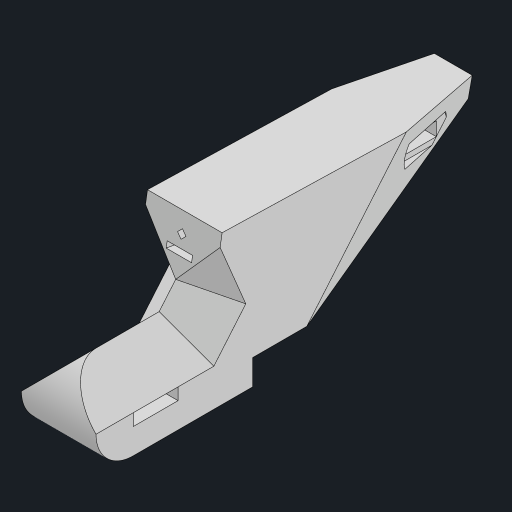
# Autodesk Inventor part: om_Body_2.0
Saved by Autodesk Inventor 2023 (Build 270158000, 158)
## iProperties
Created: 2022-06-16
Part Number: om_Body_2.0
Material: 一般
Document SubType Name: Modeling
Designer: legot
Density: 1 g/cm^3
Appearance: 既定
Mass: 644.355 g
Surface Area: 645.321 cm^2
Volume: 644.355 cm^3
Author: legot
Autodesk Inventor part; units mm, degrees
ref_plane "YZ Plane" through (0, 0, 0) normal (1, 0, 0) x (0, 1, 0)
ref_plane "XZ Plane" through (0, 0, 0) normal (0, 1, 0) x (-1, 0, 0)
ref_plane "XY Plane" through (0, 0, 0) normal (0, 0, 1) x (1, 0, 0)
sketch "スケッチ1" plane through (0, 0, 0) normal (1, 0, 0) x (0, 1, 0)
  line L0 (-36.4926, 6.1068) -> (-49.6929, 17.1832)
  line L1 (-49.6929, 17.1832) -> (-49.6929, 84.5055)
  arc A0 (-74.6929, 84.5055) -> (-99.6929, 59.5055) centre (-74.6929, 59.5055) ccw
  line L2 (-99.6929, 59.5055) -> (-99.6929, -20.4945)
  line L3 (-82.6929, -56.7945) -> (-19.7119, -179.9383)
  line L4 (-19.7119, -179.9383) -> (-4.7119, -179.9383)
  line L5 (-4.7119, -179.9383) -> (0, 0)
  line L6 (0, 0) -> (0, -120.6859) construction
  line L7 (-36.4926, 6.1068) -> (0, 0)
  line L8 (0, 0) -> (23.9477, 0) construction
  line L9 (0.4951, 2.9589) -> (52.2751, -5.7061)
  line L10 (52.2751, -5.7061) -> (51.78, -8.665)
  line L11 (51.78, -8.665) -> (0, 0)
  line L12 (39.9466, -3.643) -> (44.0728, 21.0141)
  line L13 (132.8385, 6.1598) -> (-44.6929, 35.8684)
  line L14 (-49.6929, 84.5055) -> (-74.6929, 84.5055)
  line L15 (-74.6929, 84.5055) -> (-74.6929, 5.5255)
  line L16 (-74.6929, 5.5255) -> (-49.1854, -15.8779)
  line L17 (-49.1854, -15.8779) -> (-36.4926, 6.1068)
  line L18 (-49.6929, 17.1832) -> (-74.6929, 5.5255)
  line L19 (0, 0) -> (0.4951, 2.9589)
  line L20 (-12.2119, -179.9383) -> (-12.2119, 2.0436)
  line L21 (-99.6929, -20.4945) -> (-82.6929, -20.4945)
  line L22 (-82.6929, -20.4945) -> (-82.6929, -56.7945)
  line L23 (-99.6929, -20.4945) -> (-99.6929, -23.5552)
  line L24 (-82.6929, -56.7945) -> (-99.6929, -23.5552)
  point P0 (-92.3706, 77.1832)
  dimension "d0" = 1.5
  dimension "d1" = 37
  dimension "d2" = 25
  dimension "d3" = 130
  dimension "d4" = 9.5
  dimension "d5" = 60
  dimension "d7" = 3
  dimension "d11" = 80
  dimension "d12" = 180
  dimension "d13" = 25
  dimension "d14" = 5
  dimension "d15" = 180
  dimension "d16" = 15
  dimension "d19" = 50
  dimension "d34" = 25
  dimension "d35" = 80
  dimension "d36" = 65
  dimension "d54" = 12.5
  dimension "d55" = 82
  dimension "d74" = 36.3
  dimension "d75" = 17
  dimension "d79" = 40
  constraints: 51 end point, 6 perpendicular, 6 vertical, 3 horizontal, 3 point on circle, 2 collinear, 2 midpoint, 2 parallel, 2 point on line, 2 tangent, 1 centre point
  measures "d0" angle of L6 L5
  measures "d1" distance of L5.end L0.start
  measures "d2" radius of A0
  measures "d3" angle of L6 L0
  measures "d4" angle of L8 L7
  measures "d5" vertical distance of point (-92.371, 77.183) L0.end
  measures "d7" distance of L9.end L10.end
  measures "d11" distance of L2.start L2.end
  measures "d12" distance of L13.start L13.end
  measures "d13" distance of L12.start L12.end
  measures "d14" distance from line of L13.end L1
  measures "d15" distance of L4.end L5.end
  measures "d16" distance of L3.end L4.end
  measures "d19" distance between parallel lines of L1 L2
  measures "d34" distance between parallel lines of L0 L16
  measures "d35" angle of L17 L16
  measures "d36" angle of L18 L15
  measures "d54" distance from line of L10.end L12
  measures "d55" angle of L5 L11
  measures "d74" distance of L21.end L3.start
  measures "d75" distance of L2.end L21.end
  measures "d79" distance from line of L9.start L12
extrude "押し出し1" add sketch "スケッチ1" along normal mid plane 50 contours L7 L20 L4 L3 L22 L21 L2 A0 L15 L16 L17 | L7 L5 L4 L20
ref_plane "作業平面1" through (0, -74.6929, 84.5055) normal (0, 0, 1) x (1, 0, 0)
ref_plane "作業平面3" through (0, -74.6929, 5.5255) normal (0, -0.7660444, 0.6427876) x (1, 0, 0)
sketch "スケッチ5" plane through (0, -74.6929, 5.5255) normal (0, -0.7660444, 0.6427876) x (1, 0, 0)
  line L0 (-25, 0) -> (0, 25)
  line L1 (25, 0) -> (-25, 0)
  line L2 (0, 25) -> (25, 0)
  point P0 (0, 43.7789)
  constraints: 6 end point, 1 coincident, 1 horizontal
extrude "押し出し5" add sketch "スケッチ5" against normal up to surface surface through (0, -36.4926, 6.1068) normal (0, -0.8660254, 0.5)
sketch "スケッチ6" plane through (0, -74.6929, 84.5055) normal (0, 0, 1) x (1, 0, 0)
  line L0 (25, 0) -> (-25, 0) projected
  line L1 (-25, 0) -> (0, 25)
  line L2 (0, 25) -> (25, 0)
  line L3 (25, 0) -> (-25, 0)
  point P0 (0, 74.6929)
  constraints: 6 end point, 1 collinear, 1 perpendicular
extrude "押し出し6" add sketch "スケッチ6" against normal through all
sketch "おでこ" plane through (-25, 0, 0) normal (0, 0.1650476, 0.9862856) x (1, 0, 0)
  line L0 (25, -37) -> (50, -37) projected
  line L1 (50, 0) -> (50, -37) projected
  line L2 (0, 0) -> (50, 0) projected
  line L3 (0, -37) -> (0, 0) projected
  line L4 (0, -37) -> (25, -37) projected
  line L5 (25, -37) -> (50, -8)
  line L6 (50, 10.2569) -> (50, 0) projected
  line L7 (25, -37) -> (0, -8)
  point P0 (25, 0)
  dimension "d41" = 8
  constraints: 4 end point, 2 point on line, 1 horizontal alignment
  measures "d41" distance from line of L2 L5.end
ref_plane "作業平面4" through (-1.254, -35.8559, 7.2095) normal (0.5248475, -0.3272527, 0.785774) x (0.7016738, -0.3562491, -0.6170416)
sketch "スケッチ8" plane through (-1.254, -35.8559, 7.2095) normal (0.5248475, -0.3272527, 0.785774) x (0.7016738, -0.3562491, -0.6170416)
  line L0 (1.7872, 0) -> (37.4163, 0) projected
  line L1 (1.7872, 0) -> (12.0929, 36.8754) projected
  line L2 (19.329, 12.0465) -> (37.4163, 0) projected
  line L3 (37.4163, 0) -> (12.0929, 36.8754)
  point P0 (-7.4452, 31.6782)
  constraints: 2 end point
extrude "押し出し7" cut sketch "スケッチ8" along normal blind 15
ref_plane "作業平面5" through (-11.0546, -42.1052, -3.6145) normal (-0.5248475, -0.3272527, 0.785774) x (0.7016738, 0.3562491, 0.6170416)
sketch "スケッチ9" plane through (-11.0546, -42.1052, -3.6145) normal (-0.5248475, -0.3272527, 0.785774) x (0.7016738, 0.3562491, 0.6170416)
  line L0 (15.7547, 0) -> (5.449, 36.8754) projected
  line L1 (-19.8744, 0) -> (15.7547, 0) projected
  line L2 (-19.8744, 0) -> (-1.7872, 12.0465) projected
  line L3 (-19.8744, 0) -> (5.449, 36.8754)
  point P0 (24.987, 31.6782)
  constraints: 2 end point
extrude "押し出し8" cut sketch "スケッチ9" along normal blind 15
sketch "スケッチ10" plane through (0, 0, 0) normal (1, 0, 0) x (0, 1, 0)
  arc A0 (-74.6929, 84.5055) -> (-99.6929, 59.5055) centre (-74.6929, 59.5055) ccw projected
  arc A1 (-74.6929, 84.5055) -> (-99.6929, 59.5055) centre (-74.6929, 59.5055) ccw projected
  circle A2 centre (-74.6929, 59.5055) radius 25
  line L0 (-74.6929, 5.5255) -> (-49.6929, 17.1832) projected
  line L1 (-74.6929, 84.5055) -> (-74.6929, 5.5255) projected
  line L2 (-49.6929, 84.5055) -> (-74.6929, 84.5055) projected
  line L3 (-49.6929, 84.5055) -> (-49.6929, 17.1832) projected
  point P0 (0, 0)
  point P1 (-49.6929, 59.5055)
  constraints: 1 centre point, 1 coincident, 1 concentric
extrude "押し出し9" cut sketch "スケッチ10" along normal through all both and the other way through all contours L2 L3 A2
ref_plane "作業平面9" through (25, -82.6929, -56.7945) normal (0, -0.7660444, 0.6427876) x (1, 0, 0)
sketch "スケッチ16" plane through (25, -82.6929, -56.7945) normal (0, -0.7660444, 0.6427876) x (1, 0, 0)
  line L0 (-50, -53.8502) -> (0, -53.8502) projected
  line L1 (0, 0) -> (0, -53.8502) projected
  line L2 (-50, -53.8502) -> (-50, 0) projected
  line L3 (-50, 0) -> (-35, -53.8502)
  line L4 (-15, -53.8502) -> (0, 0)
  line L5 (-35, -53.8502) -> (-15, -53.8502)
  point P0 (-25, 96.6611)
  point P1 (-25, -53.8502)
  dimension "d76" = 20
  constraints: 6 end point, 2 midpoint, 2 point on line, 1 collinear
  measures "d76" distance of L3.end L4.start
extrude "押し出し16" cut sketch "スケッチ16" against normal through all
ref_plane "作業平面11" through (12.6839, -4.7119, -179.9383) normal (0, 0, -1) x (-1, 0, 0)
sketch "スケッチ12" plane through (12.6839, -4.7119, -179.9383) normal (0, 0, -1) x (-1, 0, 0)
  line L0 (12.6839, -4.6716) -> (9.8555, -7.5)
  line L1 (9.8555, -7.5) -> (12.6839, -10.3284)
  line L2 (12.6839, -10.3284) -> (15.5123, -7.5)
  line L3 (15.5123, -7.5) -> (12.6839, -4.6716)
  line L4 (12.6839, -44.9811) -> (-12.3161, -69.9811) projected
  line L5 (25.3696, 0) -> (-0.0018, 0) projected
  line L6 (22.6839, -15) -> (25.3696, 0) projected
  line L7 (25.3696, 0) -> (-0.0018, 0) projected
  line L8 (-0.0018, 0) -> (2.6839, -15) projected
  line L9 (22.6839, -15) -> (2.6839, -15) projected
  point P0 (12.6839, 0)
  point P1 (1.341, -7.5)
  point P2 (1.341, -7.5)
  dimension "d51" = 4
  constraints: 8 end point, 2 midpoint, 2 parallel, 2 perpendicular, 2 vertical alignment, 1 coincident, 1 horizontal alignment
  measures "d51" distance of L1.end L2.end
extrude "押し出し11" cut sketch "スケッチ12" against normal through all contours L3 L2 L1 L0
sketch "スケッチ13" plane through (0, 0, 0) normal (1, 0, 0) x (0, 1, 0)
  line L0 (-39.6225, -3.5085) -> (-44.2438, -31.1245)
  line L1 (-44.2438, -31.1245) -> (-17.6141, -35.5808)
  line L2 (-17.6141, -35.5808) -> (-12.9928, -7.9648)
  line L3 (-39.6225, -3.5085) -> (-44.2438, -31.1245)
  line L4 (-44.2438, -31.1245) -> (-32.4084, -33.1051)
  line L5 (-32.4084, -33.1051) -> (-27.787, -5.4891)
  line L6 (-29.6206, -43.7107) -> (-17.9947, 25.763) construction
  line L7 (-16.0221, 25.4329) -> (-19.9672, 26.0931)
  line L8 (-19.9672, 26.0931) -> (-31.5931, -43.3806)
  line L9 (-31.5931, -43.3806) -> (-27.648, -44.0408)
  line L10 (-27.648, -44.0408) -> (-16.0221, 25.4329)
  line L11 (-12.9928, -7.9648) -> (-39.6225, -3.5085)
  line L12 (-7.8903, 1.3204) -> (-36.4926, 6.1068) projected
  point P0 (0, 0)
  point P1 (-49.6929, 17.1832)
  point P2 (-42.3628, -27.6801)
  point P3 (-41.9331, -17.3165)
  point P4 (-25.9975, -34.1779)
  point P5 (-21.3762, -6.5619)
  dimension "d56" = 27
  dimension "d57" = 28
  dimension "d66" = 4
  dimension "d67" = 10
  dimension "d70" = 12
  dimension "d71" = 4.5
  dimension "d72" = 15
  dimension "d73" = 10
  constraints: 24 end point, 6 parallel, 3 midpoint, 2 perpendicular, 2 point on line
  measures "d56" distance of L2.end L0.start
  measures "d57" distance of L0.start L0.end
  measures "d66" distance of L7.start L7.end
  measures "d67" distance between parallel lines of L9 L1
  measures "d70" distance from line of point (-41.933, -17.317) L5
  measures "d71" distance between parallel lines of L6 L5
  measures "d72" distance from line of L6 L12.end
  measures "d73" distance between parallel lines of L12 L11
extrude "押し出し12" cut sketch "スケッチ13" along normal mid plane 9.2 contours L11 L5 L1 L0
extrude "押し出し13" cut sketch "スケッチ13" along normal mid plane 26 contours L11 L8 L1 L5 | L11 L10 L1 L8 | L11 L2 L1 L10
extrude "押し出し15" cut sketch "スケッチ13" along normal mid plane 17 contours L11 L10 L1 L8 | L8 L12 L10 L11 | L1 L10 L9 L8 | L8 L7 L10 L12
sketch "スケッチ20" plane through (0, 0, 0) normal (1, 0, 0) x (0, 1, 0)
  arc A0 (-74.6929, 84.5055) -> (-99.6929, 59.5055) centre (-74.6929, 59.5055) ccw projected
  line L0 (-74.6929, 59.5055) -> (-82.6929, 59.5055)
  line L1 (-82.6929, 59.5055) -> (-82.6929, 29.5055)
  line L2 (-82.6929, 29.5055) -> (-74.6929, 29.5055)
  line L3 (-74.6929, 29.5055) -> (-74.6929, 59.5055)
  line L4 (-17.6113, -133.3893) -> (-26.8113, -133.3893)
  line L5 (-26.8113, -133.3893) -> (-26.8113, -154.3893)
  line L6 (-26.8113, -154.3893) -> (-17.6113, -154.3893)
  line L7 (-17.6113, -154.3893) -> (-17.6113, -133.3893)
  point P0 (0, 0)
  dimension "d95" = 8
  dimension "d96" = 30
  dimension "d97" = 9.2
  dimension "d98" = 21
  constraints: 16 end point, 4 parallel, 2 horizontal, 2 perpendicular
  measures "d95" distance of L0.start L0.end
  measures "d96" distance of L2.end L0.start
  measures "d97" distance of L4.start L4.end
  measures "d98" distance of L6.end L4.start
extrude "貫通" cut sketch "スケッチ20" along normal through all both and the other way through all
sketch "スケッチ21" plane through (0, 0, 0) normal (1, 0, 0) x (0, 1, 0)
  line L0 (-42.4649, -20.4945) -> (-75.6929, -20.4945)
  line L1 (-75.6929, -20.4945) -> (-75.6929, -56.7945)
  line L2 (-75.6929, -56.7945) -> (-48.5395, -56.7945)
  line L3 (-48.5395, -56.7945) -> (-42.4649, -20.4945)
  line L4 (-82.6929, -56.7945) -> (-19.7119, -179.9383) projected
  line L5 (-82.6929, -56.7945) -> (-48.5395, -56.7945)
  line L6 (-57.1208, -56.7945) -> (-57.1208, -106.7945)
  line L7 (-82.6929, -56.7945) -> (-82.6929, -20.4945) projected
  line L8 (-44.2438, -31.1245) -> (-39.6225, -3.5085) projected
  point P0 (0, 0)
  dimension "d101" = 50
  dimension "d116" = 7
  constraints: 12 end point, 3 point on line, 2 horizontal, 2 perpendicular, 1 collinear, 1 horizontal alignment, 1 parallel
  measures "d101" distance of L6.start L6.end
  measures "d116" distance between parallel lines of L1 L7
extrude "25mm" cut sketch "スケッチ21" along normal mid plane 25
sketch "スケッチ22" plane through (0, 0, 0) normal (1, 0, 0) x (0, 1, 0)
  line L0 (-82.6929, -56.7945) -> (-82.6929, -20.4945) projected
  line L1 (-75.6929, -33.6445) -> (-82.6929, -33.6445)
  line L2 (-82.6929, -33.6445) -> (-82.6929, -43.6445)
  line L3 (-82.6929, -43.6445) -> (-75.6929, -43.6445)
  line L4 (-75.6929, -43.6445) -> (-75.6929, -33.6445)
  line L5 (-75.6929, -56.7945) -> (-75.6929, -20.4945) projected
  line L6 (-42.4649, -20.4945) -> (-48.5395, -56.7945) projected
  line L7 (-47.3825, -49.8804) -> (-23.6929, -133.3893)
  line L8 (-48.5395, -56.7945) -> (-26.8113, -133.3893)
  line L9 (-17.6113, -133.3893) -> (-26.8113, -133.3893) projected
  point P0 (0, 0)
  point P1 (-82.6929, -38.6445)
  point P2 (-39.6292, -3.5488)
  dimension "d106" = 10
  dimension "d110" = 3
  constraints: 11 end point, 4 point on line, 2 horizontal, 2 midpoint, 2 parallel, 1 horizontal alignment, 1 perpendicular, 3 other
  measures "d106" distance of L4.start L1.start
  measures "d110" distance between parallel lines of L7 L8
extrude "配線（3mm）" cut sketch "スケッチ22" along normal mid plane 3
ref_plane "作業平面12" through (14.1806, -26.8113, -154.3893) normal (1, 0, 0) x (0, 0, -1)
sketch "スケッチ24" plane through (14.1806, -26.8113, -154.3893) normal (1, 0, 0) x (0, 0, -1)
  line L0 (-21, 0) -> (-21, 9.2) projected
  line L1 (-21, 9.2) -> (0, 9.2) projected
  line L2 (0, 9.2) -> (0, 0) projected
  line L3 (0, 0) -> (-21, 0) projected
  line L4 (25.549, 7.0994) -> (-97.5948, -55.8817) projected
  line L5 (25.549, 22.0994) -> (25.549, 7.0994) projected
  line L6 (-30.9201, 23.5781) -> (25.549, 22.0994) projected
  line L7 (-97.5948, -55.8817) -> (-30.9201, 23.5781) projected
  circle A0 centre (-10.5, 4.6) radius 17.5
  line L8 (-26, 12.724) -> (5, 12.724)
  line L9 (-26, -3.524) -> (5, -3.524)
  point P0 (-154.3893, 26.8113)
  point P1 (-21, 4.6)
  point P2 (-10.5, 9.2)
  point P3 (4.7775, -3.524)
  point P4 (5.0802, -3.3692)
  dimension "d117" = 35
  dimension "d118" = 31
  constraints: 4 end point, 4 point on circle, 2 midpoint, 2 parallel, 1 centre point, 1 horizontal, 1 horizontal alignment, 1 vertical alignment
  measures "d117" diameter of A0
  measures "d118" distance of L9.start L9.end
extrude "押し出し24" cut sketch "スケッチ24" along normal through all contours L4 L9 A0 L8
ref_plane "作業平面13" through (-14.1806, -26.8113, -154.3893) normal (-1, 0, 0) x (0, 0, 1)
sketch "スケッチ25" plane through (-14.1806, -26.8113, -154.3893) normal (-1, 0, 0) x (0, 0, 1)
  circle A0 centre (10.5, 4.6) radius 17.5 projected
  line L0 (26, -3.524) -> (-5, -3.524) projected
  line L1 (26, 12.724) -> (-5, 12.724) projected
  line L2 (21, 9.2) -> (0, 9.2) projected
  line L3 (21, 9.2) -> (21, 0) projected
  line L4 (0, 0) -> (21, 0) projected
  line L5 (0, 9.2) -> (0, 0) projected
  point P0 (154.3893, 26.8113)
extrude "押し出し25" cut sketch "スケッチ25" along normal through all contours A0 L0 L1
sketch "スケッチ14" plane through (0, 0, 0) normal (1, 0, 0) x (0, 1, 0)
  line L0 (51.7239, 145.6889) -> (-136.8332, 145.6889)
  line L1 (-136.8332, 145.6889) -> (-136.8332, -201.0178)
  line L2 (-136.8332, -201.0178) -> (51.7239, -201.0178)
  line L3 (51.7239, -201.0178) -> (51.7239, 145.6889)
  point P0 (0, 0)
  constraints: 8 end point, 2 parallel, 1 horizontal, 1 perpendicular
extrude "右半分" [suppressed]
